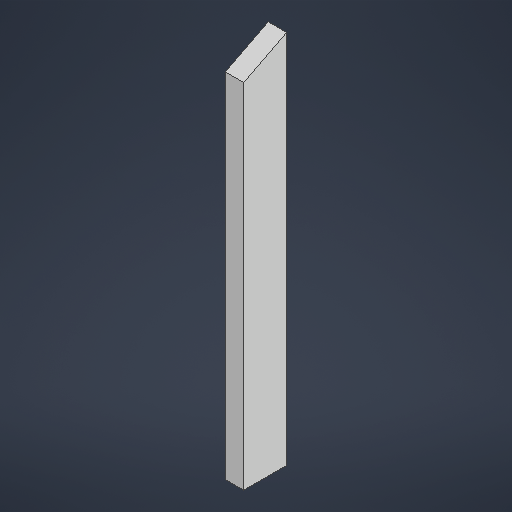
# Autodesk Inventor part: S_2x4x30.5
Saved by Autodesk Inventor 2027.1 (Build 311270010, 270A)
## iProperties
Created: 2026-09-01
Part Number: S_2x4x30.5
Material: Generic
Document SubType Name: Modeling
Designer: jorda
Density: 1 g/cm^3
Appearance: Default
Author: jorda
Autodesk Inventor part; units mm, degrees
ref_plane "YZ Plane" through (0, 0, 0) normal (1, 0, 0) x (0, 1, 0)
ref_plane "XZ Plane" through (0, 0, 0) normal (0, 1, 0) x (-1, 0, 0)
ref_plane "XY Plane" through (0, 0, 0) normal (0, 0, 1) x (1, 0, 0)
sketch "Sketch1" plane through (0, 0, 0) normal (1, 0, 0) x (0, 1, 0)
  line L0 (0, 0) -> (709.2052, 0)
  line L1 (774.7, -88.9) -> (0, -88.9)
  line L2 (0, -88.9) -> (0, 0)
  line L3 (774.7, -88.9) -> (909.5108, -88.9) construction
  line L4 (774.7, -88.9) -> (729.4486, 0)
  line L5 (729.4486, 0) -> (709.2052, 0)
  constraints: 12 end point, 3 horizontal, 1 parallel
extrude "Extrusion1" add sketch "Sketch1" along normal blind 38.1
body "Solid1"
